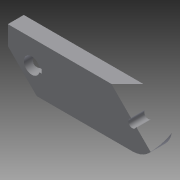
# Autodesk Inventor part: arm
Saved by Autodesk Inventor 2015 SP1 (Build 190203100, 203)
## iProperties
Created: 2016-02-02
Part Number: arm
Material: Generic
Document SubType Name: Modeling
Designer: tuttlem
Density: 1 g/cm^3
Appearance: Default
Author: tuttlem
Autodesk Inventor part; units mm, degrees
ref_plane "YZ Plane" through (0, 0, 0) normal (1, 0, 0) x (0, 1, 0)
ref_plane "XZ Plane" through (0, 0, 0) normal (0, 1, 0) x (-1, 0, 0)
ref_plane "XY Plane" through (0, 0, 0) normal (0, 0, 1) x (1, 0, 0)
sketch "Sketch1" plane through (0, 0, 0) normal (0, 0, 1) x (1, 0, 0)
  line L0 (-99.06, 38.1) -> (-99.06, -38.1)
  circle A0 centre (-60.96, 0) radius 12.7
  circle A1 centre (99.06, 0) radius 6.35
  line L1 (-99.06, 38.1) -> (99.06, 38.1)
  line L2 (-99.06, -38.1) -> (99.06, -38.1)
  arc A2 (99.06, -38.1) -> (99.06, 38.1) centre (99.06, 0) ccw
  line L3 (-48.6633, 3.175) -> (-45.3613, 3.175)
  line L4 (-45.3613, 3.175) -> (-45.3613, -3.175)
  line L5 (-45.3613, -3.175) -> (-48.6633, -3.175)
  point P0 (0, 0)
  point P1 (-99.06, 0)
  point P2 (106.7321, -3.216)
  point P3 (113.0654, -3.216)
  point P4 (-45.3613, 0)
  point P5 (0, -38.1)
  dimension "d0" = 76.2
  dimension "d4" = 25.4
  dimension "d13" = 12.7
  dimension "d14" = 6.35
  dimension "d15" = 160.02
  dimension "d16" = 3.302
  dimension "d17" = 38.1
  constraints: 12 end point, 4 horizontal alignment, 4 point on circle, 3 centre point, 3 midpoint, 2 horizontal, 2 perpendicular, 2 vertical alignment, 1 coincident, 1 parallel, 1 vertical
  measures "d0" distance of L0.start L0.end
  measures "d4" diameter of A0
  measures "d13" diameter of A1
  measures "d14" distance of L3.end L4.end
  measures "d15" distance of A1.centre A0.centre
  measures "d16" distance of L4.end L5.end
  measures "d17" distance from line of A0.centre L0
extrude "Extrusion2" add sketch "Sketch1" along normal blind 25.4
body "Solid2"
